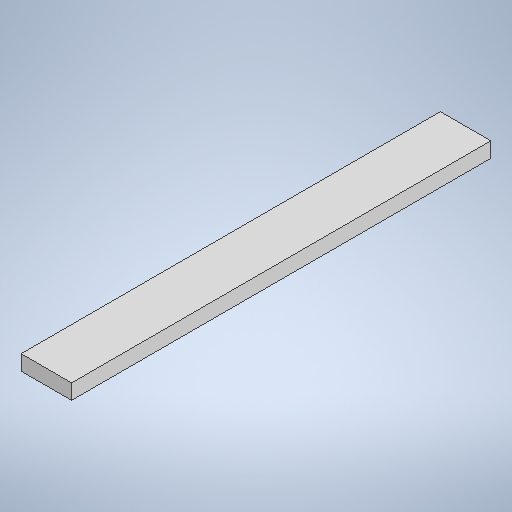
# Autodesk Inventor part: Probe_Platzhalter
Saved by Autodesk Inventor 2025 (Build 290162000, 162)
## iProperties
Created: 2026-07-01
Part Number: Probe_Platzhalter
Material: Generisch
Document SubType Name: Modeling
Designer: wavid
Mass: 19.92 g
Surface Area: 88.72 cm^2
Volume: 19.92 cm^3
Density: 1 g/cm^3
Appearance: Vorgabe
Author: wavid
Autodesk Inventor part; units mm, degrees
ref_plane "YZ Plane" through (0, 0, 0) normal (1, 0, 0) x (0, 1, 0)
ref_plane "XZ Plane" through (0, 0, 0) normal (0, 1, 0) x (-1, 0, 0)
ref_plane "XY Plane" through (0, 0, 0) normal (0, 0, 1) x (1, 0, 0)
sketch "Skizze1" plane through (0, 0, 0) normal (0, 0, 1) x (1, 0, 0)
  line L0 (-10, -83) -> (10, -83)
  line L1 (10, -83) -> (10, 83)
  line L2 (10, 83) -> (-10, 83)
  line L3 (-10, 83) -> (-10, -83)
  constraints: 8 end point, 2 parallel, 1 horizontal, 1 perpendicular
extrude "Extrusion1" add sketch "Skizze1" along normal blind 6
